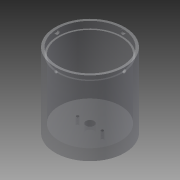
# Autodesk Inventor part: 13_1087_060
Saved by Autodesk Inventor 2014 SP1 (Build 180222100, 222)
## iProperties
Created: 2013-12-09
Part Number: 13_1087_060
Material: Allgemein
Document SubType Name: Modeling
Designer: vogel
Density: 1 g/cm^3
Appearance: Polycarbonat - klar
Author: vogel
Autodesk Inventor part; units mm, degrees
ref_plane "YZ Plane" through (0, 0, 0) normal (1, 0, 0) x (0, 1, 0)
ref_plane "XY Plane" through (0, 0, 0) normal (0, 0, 1) x (1, 0, 0)
sketch "Skizze1" plane through (0, 0, 0) normal (0, 0, 1) x (1, 0, 0)
  line L0 (-29.4, 0) -> (29.4, 0) projected
  line L1 (0, -29.4) -> (0, 29.4) projected
  circle A0 centre (0, 0) radius 21
  dimension "d0" = 42
  constraints: 1 centre point, 1 coincident
  measures "d0" diameter of A0
extrude "Extrusion1" add sketch "Skizze1" along normal blind 5
sketch "Skizze2" plane through (0, 0, 5) normal (0, 0, 1) x (1, 0, 0)
  circle A0 centre (0, 0) radius 21 projected
  circle A1 centre (0, 0) radius 21
  circle A2 centre (0, 0) radius 19.5
  dimension "d3" = 39
  constraints: 2 centre point, 2 coincident, 1 concentric
  measures "d3" diameter of A2
extrude "Extrusion2" add sketch "Skizze2" along normal blind 40
sketch "Skizze3" plane through (0, 0, 0) normal (0, 0, -1) x (-1, 0, 0)
  line L0 (29.4, 0) -> (-29.4, 0) projected
  line L1 (0, -29.4) -> (0, 29.4) projected
  point P0 (-7.5, 0)
  point P1 (7.5, 0)
  dimension "d6" = 15
  constraints: 2 point on line, 1 symmetric about line
  measures "d6" distance of point (7.5, 0) point (-7.5, 0)
hole "Bohrung1" at (7.5, 0, 0) at (-7.5, 0, 0) direction (0, 0, 1) diameter 1.567 end through all thread size "M2x0.4" class "6H" standard "ISO Metric profile"
hole "Bohrung2" at (0, 0, 0) direction (0, 0, 1) diameter 5 end through all
ref_plane "Arbeitsebene1" through (0, -21, 0) normal (0, 1, 0) x (-1, 0, 0)
sketch "Skizze4" plane through (0, -21, 0) normal (0, 1, 0) x (-1, 0, 0)
  line L0 (29.4, 0) -> (-29.4, 0) projected
  line L1 (0, -9) -> (0, 54) projected
  line L2 (21, 45) -> (-21, 45) projected
  point P0 (0, 0)
  point P1 (0, 43)
  dimension "d23" = 2
  constraints: 1 point on line
  measures "d23" distance from line of point (0, 43) L2
hole "Bohrung3" at (0, -21, 43) direction (0, 1, 0) diameter 2.4 end through all
pattern_circular "Runde Anordnung1" count 4 over 360 about axis through (0, 0, -10) along (0, 0, 1) of "Bohrung3"
sketch "Skizze5" plane through (0, 0, 5) normal (0, 0, 1) x (1, 0, 0)
  circle A0 centre (0, 0) radius 19.5 projected
  circle A1 centre (0, 0) radius 18.5
  dimension "d34" = 37
  constraints: 1 centre point, 1 coincident
  measures "d34" diameter of A1
extrude "Extrusion3" add sketch "Skizze5" along normal blind 36
